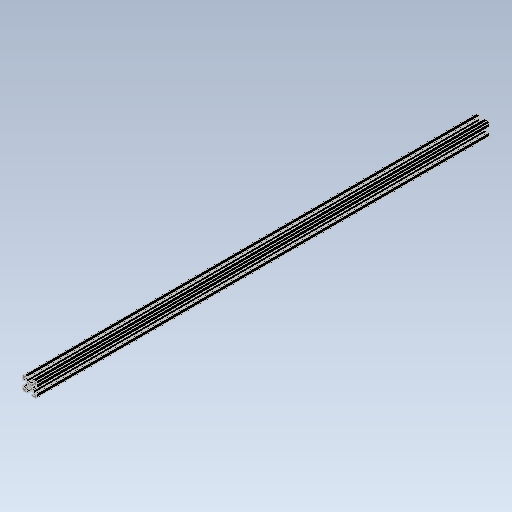
# Autodesk Inventor part: ITEM_20x20_630mm
Saved by Autodesk Inventor 2021 (Build 250183000, 183)
## iProperties
Part Number: ITEM_20x20_630mm
Material: Generic
Document SubType Name: Modeling
Designer: Alexander Fritzsche
Appearance: Default
Author: Alexander Fritzsche
Autodesk Inventor part; units mm, degrees
ref_plane "YZ Plane" through (0, 0, 0) normal (1, 0, 0) x (0, 1, 0)
ref_plane "XZ Plane" through (0, 0, 0) normal (0, 1, 0) x (-1, 0, 0)
ref_plane "XY Plane" through (0, 0, 0) normal (0, 0, 1) x (1, 0, 0)
sketch "Sketch1" plane through (0, 0, 0) normal (0, 0, 1) x (1, 0, 0)
  circle A0 centre (0, 0) radius 2.15
  line L0 (-10, 10) -> (-2.5, 10)
  line L1 (-2.5, 10) -> (-2.5, 8.2)
  line L2 (-2.5, 8.2) -> (-6.9272, 8.2)
  line L3 (-6.9272, 8.2) -> (-2.3772, 3.65)
  line L4 (-2.3772, 3.65) -> (2.3772, 3.65)
  line L5 (2.3772, 3.65) -> (6.9272, 8.2)
  line L6 (6.9272, 8.2) -> (2.5, 8.2)
  line L7 (2.5, 8.2) -> (2.5, 10)
  line L8 (2.5, 10) -> (10, 10)
  line L9 (10, 10) -> (10, 2.5)
  line L10 (10, 2.5) -> (8.2, 2.5)
  line L11 (8.2, 2.5) -> (8.2, 6.9272)
  line L12 (8.2, 6.9272) -> (3.65, 2.3772)
  line L13 (3.65, 2.3772) -> (3.65, -2.3772)
  line L14 (3.65, -2.3772) -> (8.2, -6.9272)
  line L15 (8.2, -6.9272) -> (8.2, -2.5)
  line L16 (8.2, -2.5) -> (10, -2.5)
  line L17 (10, -2.5) -> (10, -10)
  line L18 (10, -10) -> (2.5, -10)
  line L19 (2.5, -10) -> (2.5, -8.2)
  line L20 (2.5, -8.2) -> (6.9272, -8.2)
  line L21 (6.9272, -8.2) -> (2.3772, -3.65)
  line L22 (2.3772, -3.65) -> (-2.3772, -3.65)
  line L23 (-2.3772, -3.65) -> (-6.9272, -8.2)
  line L24 (-6.9272, -8.2) -> (-2.5, -8.2)
  line L25 (-2.5, -8.2) -> (-2.5, -10)
  line L26 (-2.5, -10) -> (-10, -10)
  line L27 (-10, -10) -> (-10, -2.5)
  line L28 (-10, -2.5) -> (-8.2, -2.5)
  line L29 (-8.2, -2.5) -> (-8.2, -6.9272)
  line L30 (-8.2, -6.9272) -> (-3.65, -2.3772)
  line L31 (-3.65, -2.3772) -> (-3.65, 2.3772)
  line L32 (-3.65, 2.3772) -> (-8.2, 6.9272)
  line L33 (-8.2, 6.9272) -> (-8.2, 2.5)
  line L34 (-8.2, 2.5) -> (-10, 2.5)
  line L35 (-10, 2.5) -> (-10, 10)
  line L36 (0, 0) -> (-30.8654, 30.8654)
  line L37 (0, 0) -> (30.8654, 30.8654)
  line L38 (0, 0) -> (42.5392, 0)
  line L39 (0, 0) -> (0, 44.3419)
  dimension "d0" = 45
  dimension "d1" = 90
  dimension "Breite" = 20
  dimension "Tiefe_Schiene" = 6.35
  dimension "d2" = 1.8
  dimension "Durchmesser_Loch" = 4.3
  dimension "Wandstaerke" = 1.8
  dimension "d3" = 1.8
  dimension "Breite_Schiene" = 5
  dimension "d4" = 5
  constraints: 80 end point, 19 point on line, 17 perpendicular, 13 parallel, 7 collinear, 2 horizontal, 1 centre point, 1 coincident, 1 vertical, 8 other
  measures "d0" angle of L37 L38
  measures "d1" angle of L37 L36
  measures "Breite" distance between parallel lines of L18 L8
  measures "Tiefe_Schiene" distance between parallel lines of L8 L4
  measures "d2" distance between parallel lines of L0 L2
  measures "Durchmesser_Loch" diameter of A0
  measures "Wandstaerke" distance between parallel lines of L3 L32
  measures "d3" distance between parallel lines of L23 L30
  measures "Breite_Schiene" distance between parallel lines of L28 L34
  measures "d4" distance between parallel lines of L7 L1
extrude "Extrusion1" add sketch "Sketch1" along normal mid plane 630 contours L38 L13 L14 L15 L16 L17 L18 L19 L20 L21 L22 L23 L24 L25 L26 L27 L28 L29 L30 L31 L32 L33 L34 L35 L36 A0 | A0 L37 L9 L10 L11 L12 L13 L38 | A0 L39 L4 L5 L6 L7 L8 L37 | L36 L0 L1 L2 L3 L4 L39 A0
fillet "Fillet1" radius 2 4 edges at (10, 10, 0) (-10, 10, 0) (10, -10, 0) (-10, -10, 0)
fillet "Fillet2" radius 0.2 8 edges at (-2.5, 8.2, 0) (2.5, 8.2, 0) (8.2, 2.5, 0) (8.2, -2.5, 0) (-2.5, -8.2, 0) (-8.2, -2.5, 0) (-8.2, 2.5, 0) (2.5, -8.2, 0)
fillet "Fillet3" radius 0.7 16 edges at (-2.5, 10, 0) (2.5, 10, 0) (10, 2.5, 0) (10, -2.5, 0) (2.5, -10, 0) (-2.5, -10, 0) (-10, -2.5, 0) (-10, 2.5, 0) (-6.9272, -8.2, 0) (-8.2, -6.9272, 0) (6.9272, -8.2, 0) (8.2, -6.9272, 0) (8.2, 6.9272, 0) (6.9272, 8.2, 0) (-6.9272, 8.2, 0) (-8.2, 6.9272, 0)
fillet "Fillet4" radius 2 8 edges at (-3.65, 2.3772, 0) (-2.3772, 3.65, 0) (2.3772, 3.65, 0) (3.65, 2.3772, 0) (3.65, -2.3772, 0) (2.3772, -3.65, 0) (-2.3772, -3.65, 0) (-3.65, -2.3772, 0)
equation "\"d2\" = Wandstaerke"
equation "\"d3\" = Wandstaerke"
equation "\"d4\" = Breite_Schiene"
body "Solid1"
